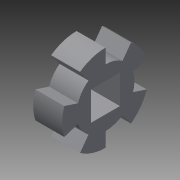
# Autodesk Inventor part: SmallGear
Saved by Autodesk Inventor 2015 (Build 190159000, 159)
## iProperties
Created: 2015-06-16
Part Number: SmallGear
Material: Generic
Document SubType Name: Modeling
Designer: david_000
Density: 1 g/cm^3
Appearance: Default
Author: david_000
Autodesk Inventor part; units mm, degrees
ref_plane "YZ Plane" through (0, 0, 0) normal (1, 0, 0) x (0, 1, 0)
ref_plane "XZ Plane" through (0, 0, 0) normal (0, 1, 0) x (-1, 0, 0)
ref_plane "XY Plane" through (0, 0, 0) normal (0, 0, 1) x (1, 0, 0)
sketch "Sketch1" plane through (0, 0, 0) normal (1, 0, 0) x (0, 1, 0)
  line L0 (0, 0) -> (1.27, 0)
  line L1 (1.27, 0) -> (1.27, -1.27)
  line L2 (1.27, -1.27) -> (0, -1.27)
  line L3 (0, -1.27) -> (0, 0)
  arc A0 (0.2425, 0.5728) -> (-0.3925, 0.1115) centre (0.635, -0.635) ccw
  line L4 (-0.3925, 0.1115) -> (-0.9062, 0.4847)
  line L5 (-0.635, -0.635) -> (-1.27, -0.635)
  arc A1 (-0.9062, 0.4847) -> (-1.27, -0.635) centre (0.635, -0.635) ccw
  line L6 (-0.635, -0.635) -> (-1.27, -0.635)
  line L7 (-0.3925, -1.3815) -> (-0.9062, -1.7547)
  line L8 (0.2425, -1.8428) -> (0.0463, -2.4468)
  line L9 (1.0275, -1.8428) -> (1.2237, -2.4468)
  line L10 (1.6625, -1.3815) -> (2.1762, -1.7547)
  line L11 (1.905, -0.635) -> (2.54, -0.635)
  line L12 (1.6625, 0.1115) -> (2.1762, 0.4847)
  line L13 (1.0275, 0.5728) -> (1.2237, 1.1768)
  line L14 (0.2425, 0.5728) -> (0.0463, 1.1768)
  arc A2 (0.2425, 0.5728) -> (-0.3925, 0.1115) centre (0.635, -0.635) ccw
  arc A3 (1.6625, 0.1115) -> (1.0275, 0.5728) centre (0.635, -0.635) ccw
  arc A4 (1.6625, -1.3815) -> (1.905, -0.635) centre (0.635, -0.635) ccw
  arc A5 (-0.635, -0.635) -> (-0.3925, -1.3815) centre (0.635, -0.635) ccw
  arc A6 (0.2425, -1.8428) -> (1.0275, -1.8428) centre (0.635, -0.635) ccw
  arc A7 (1.2237, 1.1768) -> (0.0463, 1.1768) centre (0.635, -0.635) ccw
  arc A8 (2.54, -0.635) -> (2.1762, 0.4847) centre (0.635, -0.635) ccw
  arc A9 (-0.9062, -1.7547) -> (0.0463, -2.4468) centre (0.635, -0.635) ccw
  arc A10 (1.2237, -2.4468) -> (2.1762, -1.7547) centre (0.635, -0.635) ccw
  dimension "d0" = 1.27
  dimension "d1" = 1.27
  dimension "d9" = 360
  constraints: 30 end point, 22 point on circle, 11 centre point, 2 coincident, 2 horizontal, 2 parallel, 1 perpendicular, 31 other
  measures "d0" distance of L1.end L2.end
  measures "d1" distance of L0.end L1.end
extrude "Extrusion1" add sketch "Sketch1" along normal blind 1.27
body "Solid1"
